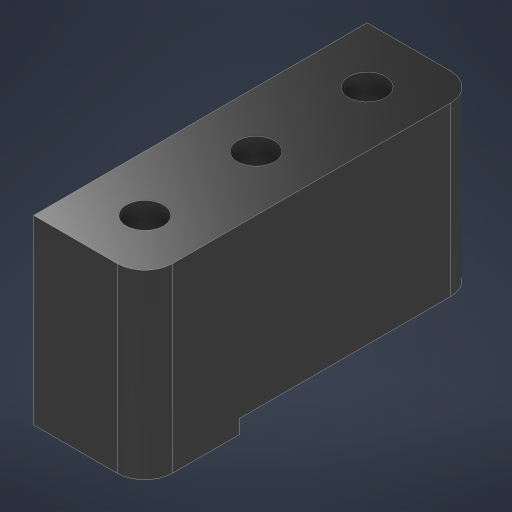
# Autodesk Inventor part: inner wing mount
Saved by Autodesk Inventor 2024 (Build 280153000, 153)
## iProperties
Created: 2023-12-24
Part Number: inner wing mount
Material: Generic
Document SubType Name: Modeling
Designer: elite
Density: 1 g/cm^3
Appearance: Glossy - Black
Author: elite
Autodesk Inventor part; units mm, degrees
ref_plane "YZ Plane" through (0, 0, 0) normal (1, 0, 0) x (0, 1, 0)
ref_plane "XZ Plane" through (0, 0, 0) normal (0, 1, 0) x (-1, 0, 0)
ref_plane "XY Plane" through (0, 0, 0) normal (0, 0, 1) x (1, 0, 0)
sketch "Sketch1" plane through (0, 0, 0) normal (0, 1, 0) x (-1, 0, 0)
  line L0 (0, 0) -> (12.7, 0)
  line L1 (12.7, 0) -> (12.7, -38.1)
  line L2 (12.7, -38.1) -> (0, -38.1)
  line L3 (0, -38.1) -> (0, 0)
  line L4 (6.35, 0) -> (6.35, -6.35)
  circle A0 centre (6.35, -6.35) radius 2.1082
  line L5 (6.35, -6.35) -> (6.35, -19.05)
  line L6 (6.35, -19.05) -> (6.35, -31.75)
  circle A1 centre (6.35, -19.05) radius 2.1082
  circle A2 centre (6.35, -31.75) radius 2.1082
  dimension "d0" = 12.7
  dimension "d1" = 38.1
  dimension "d2" = 6.35
  dimension "d3" = 4.2164
  dimension "d4" = 12.7
  dimension "d5" = 12.7
  dimension "d6" = 4.2164
  dimension "d7" = 4.2164
  constraints: 14 end point, 3 centre point, 3 coincident, 2 parallel, 2 vertical, 1 horizontal, 1 midpoint, 1 perpendicular, 1 point on line
  measures "d0" distance of L1.end L2.end
  measures "d1" distance of L2.end L0.start
  measures "d2" distance of L4.start L4.end
  measures "d3" diameter of A0
  measures "d4" distance of L5.start L5.end
  measures "d5" distance of L5.end L6.end
  measures "d6" diameter of A1
  measures "d7" diameter of A2
extrude "Extrusion1" add sketch "Sketch1" along normal blind 19.1516
sketch "Sketch2" plane through (0, 0, 0) normal (0, -1, 0) x (1, 0, 0)
  circle A0 centre (-6.35, -19.05) radius 2.1082 projected
  circle A1 centre (-6.35, -19.05) radius 5.08
  point P0 (0, 0)
  dimension "d11" = 10.16
  constraints: 1 centre point, 1 coincident
  measures "d11" diameter of A1
extrude "Extrusion2" cut sketch "Sketch2" against normal blind 6.35
sketch "Sketch3" plane through (0, 0, 0) normal (0, -1, 0) x (1, 0, 0)
  line L0 (-12.7, -38.1) -> (-12.7, 0) projected
  line L1 (-12.7, 0) -> (-12.7, -10.795)
  line L2 (-12.7, -10.795) -> (0, -10.795)
  line L3 (0, 0) -> (0, -38.1) projected
  line L4 (0, 0) -> (-12.7, 0)
  point P0 (0, -3.175)
  dimension "d15" = 10.795
  constraints: 6 end point, 2 point on line, 1 parallel, 1 perpendicular
  measures "d15" distance of L0.end L1.end
extrude "Extrusion3" add sketch "Sketch3" along normal blind 1.5875
fillet "Fillet3" radius 3.175 1 edges at (0, 8.782, 0)
sketch "Sketch4" plane through (-6.35, 0, -6.35) normal (0, 1, 0) x (1, 0, 0)
  circle A0 centre (0, 0) radius 2.1082
  point P0 (6.35, -6.35)
  constraints: 1 centre point
extrude "Extrusion4" cut sketch "Sketch4" against normal blind 3.175
fillet "Fillet4" radius 3.175 1 edges at (0, 9.5758, -38.1)
body "Solid1"
